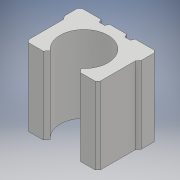
# Autodesk Inventor part: PilowBlockAbertoSBR16
Saved by Autodesk Inventor 2018 (Build 220112000, 112)
## iProperties
Created: 2018-09-20
Part Number: PilowBlockAbertoSBR16
Material: Genérico
Document SubType Name: Modeling
Designer: Georgines
Density: 1 g/cm^3
Appearance: Padrão
Author: Georgines
Autodesk Inventor part; units mm, degrees
ref_plane "YZ Plane" through (0, 0, 0) normal (1, 0, 0) x (0, 1, 0)
ref_plane "XZ Plane" through (0, 0, 0) normal (0, 1, 0) x (-1, 0, 0)
ref_plane "XY Plane" through (0, 0, 0) normal (0, 0, 1) x (1, 0, 0)
sketch "Esboço1" plane through (0, 0, 0) normal (0, 0, 1) x (1, 0, 0)
  line L0 (-22.5, 16.605) -> (22.5, 16.605) construction
  line L1 (22.5, 16.605) -> (22.5, -16.395) construction
  line L2 (22.5, -16.395) -> (-22.5, -16.395) construction
  line L3 (-22.5, -16.395) -> (-22.5, 16.605) construction
  line L4 (-14, 20.4248) -> (-14, -25.3484) construction
  line L5 (14, 20.4248) -> (14, -25.3484) construction
  line L6 (0, 20.9223) -> (0, -24.8509) construction
  line L7 (-26.3196, -3.395) -> (26.3196, -3.395) construction
  line L8 (-26.3196, 7.605) -> (26.3196, 7.605) construction
  line L9 (-21, 20.7786) -> (-21, -24.9946) construction
  line L10 (21, 20.4248) -> (21, -25.3484) construction
  line L11 (0, -3.395) -> (-21.4941, -29.0107) construction
  line L12 (0, -3.395) -> (21.8166, -29.395) construction
  line L13 (-10, 20.4248) -> (-10, -25.3484) construction
  line L14 (-5, 20.4248) -> (-5, -25.3484) construction
  line L15 (5, 20.9223) -> (5, -24.8509) construction
  line L16 (10, 20.9223) -> (10, -24.8509) construction
  line L17 (-26.3196, 5.605) -> (26.3196, 5.605) construction
  line L18 (-22.5, 16.605) -> (-22.5, 7.605)
  line L19 (-22.5, 7.605) -> (-21, 5.605)
  line L20 (-21, 5.605) -> (-21, -16.395)
  line L21 (-21, -16.395) -> (-10.9083, -16.395)
  line L22 (-10.9083, -16.395) -> (-8.999, -14.1196)
  line L23 (8.999, -14.1196) -> (10.9083, -16.395)
  line L24 (10.9083, -16.395) -> (21, -16.395)
  line L25 (22.5, 7.605) -> (22.5, 16.605)
  line L26 (26.3196, 14.605) -> (-26.3196, 14.605) construction
  line L27 (-22.5, 16.605) -> (-10, 16.605)
  line L28 (-5, 16.605) -> (5, 16.605)
  line L29 (22.5, 16.605) -> (10, 16.605)
  arc A0 (8.999, -14.1196) -> (-8.999, -14.1196) centre (0, -3.395) ccw
  line L30 (-10, 16.605) -> (-7.6714, 16.605) construction
  line L31 (-10, 16.605) -> (-9.0674, 14.605)
  line L32 (-10, 16.605) -> (-7.7932, 16.605) construction
  line L33 (-5, 16.605) -> (-5.9326, 14.605)
  line L34 (-5, 16.605) -> (-2.7932, 16.605) construction
  line L35 (-5.9326, 14.605) -> (-9.0674, 14.605)
  line L36 (5, 16.605) -> (5.9326, 14.605)
  line L37 (10, 16.605) -> (9.0674, 14.605)
  line L38 (5.9326, 14.605) -> (9.0674, 14.605)
  line L39 (21, -16.395) -> (21, 5.605)
  line L40 (22.5, 7.605) -> (21, 5.605)
  point P0 (0, 0)
  point P1 (0, 16.605)
  point P2 (0, 7.605)
  dimension "largura" = 45
  dimension "altura" = 33
  dimension "d2" = 14
  dimension "d3" = 14
  dimension "d4" = 20
  dimension "d5" = 9
  dimension "d7" = 1.5
  dimension "d8" = 1.5
  dimension "d9" = 40
  dimension "d10" = 40
  dimension "d11" = 5
  dimension "d12" = 5
  dimension "d13" = 10
  dimension "d14" = 10
  dimension "d15" = 2
  dimension "d16" = 2
  dimension "d18" = 14
  dimension "d21" = 115
  dimension "d22" = 115
  dimension "d23" = 115
  dimension "d24" = 115
  constraints: 82 end point, 32 point on line, 7 vertical, 6 horizontal, 6 parallel, 4 collinear, 4 midpoint, 2 coincident, 2 equal length, 2 point on circle, 1 centre point, 1 perpendicular
  measures "largura" distance of L0.start L0.end
  measures "altura" distance of L2.end L0.start
  measures "d2" distance between parallel lines of L4 L6
  measures "d3" distance between parallel lines of L5 L6
  measures "d4" distance between parallel lines of L7 L0
  measures "d5" distance between parallel lines of L8 L0
  measures "d7" distance between parallel lines of L1 L10
  measures "d8" distance between parallel lines of L3 L9
  measures "d9" angle of L11 L6
  measures "d10" angle of L6 L12
  measures "d11" distance between parallel lines of L14 L6
  measures "d12" distance between parallel lines of L15 L6
  measures "d13" distance between parallel lines of L13 L6
  measures "d14" distance between parallel lines of L16 L6
  measures "d15" distance between parallel lines of L17 L8
  measures "d16" distance between parallel lines of L26 L0
  measures "d18" radius of A0
  measures "d21" angle of L33 L34
  measures "d22" angle of L37 L0
  measures "d23" angle of L36 L28
  measures "d24" angle of L31 L0
extrude "Extrusão1" add sketch "Esboço1" along normal blind 45
chamfer "Chanfro1" distance 1.5 angle 45 4 edges at (22.5, 16.605, 22.5) (-22.5, 16.605, 22.5) (21, -16.395, 22.5) (-21, -16.395, 22.5)
equation "\"d3\" = d2"
equation "\"d8\" = d7"
equation "\"d10\" = d9"
equation "\"d12\" = d11"
equation "\"d14\" = d13"
